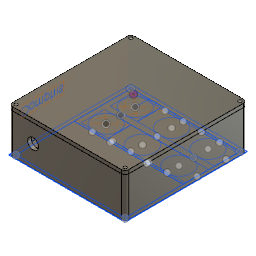
Multiple Contacts (Autodesk Fusion 360 design; units mm, degrees)
Autodesk Fusion 360 part; units mm, degrees
note: some values were not read from the file. Chosen so that the rebuilt part matches the saved one: which face or edge a step refers to; how an offset face is resized. Set by a fixed rule: which sketch regions a step uses.
sketch "Sketch1" plane through (0, 0, 0) normal (0, 1, 0) x (1, 0, 0)
  circle A0 centre (16.5, -34) radius 2.5
  line L0 (41.5, 5) -> (-8.5, 5)
  line L1 (-8.5, 5) -> (-8.5, -73)
  line L2 (-8.5, -73) -> (41.5, -73)
  line L3 (41.5, 5) -> (-8.5, -73) construction
  line L4 (-8.5, 5) -> (41.5, -73) construction
  circle A1 centre (16.5, -14) radius 17.6966
  circle A2 centre (16.5, -54.0395) radius 17.7007
  line L5 (35, 2) -> (-2, 2)
  line L6 (-2, 2) -> (-2, -30)
  line L7 (-2, -30) -> (35, -30)
  line L8 (35, -30) -> (35, 2)
  line L9 (35, 2) -> (-2, -30) construction
  line L10 (-2, 2) -> (35, -30) construction
  line L11 (35, -38.0395) -> (-2, -38.0395)
  line L12 (-2, -38.0395) -> (-2, -70.0395)
  line L13 (-2, -70.0395) -> (35, -70.0395)
  line L14 (35, -70.0395) -> (35, -38.0395)
  line L15 (35, -38.0395) -> (-2, -70.0395) construction
  line L16 (-2, -38.0395) -> (35, -70.0395) construction
  line L17 (41.5, 5) -> (91.5, 5)
  line L18 (91.5, -73) -> (41.5, -73)
  line L19 (91.5, 5) -> (141.5, 5)
  line L20 (141.5, 5) -> (141.5, -73)
  line L21 (141.5, -73) -> (91.5, -73)
  line L22 (35, 2) -> (141.5, 2)
  line L23 (141.5, 2) -> (141.5, -30)
  line L24 (141.5, -30) -> (35, -30)
  line L25 (35, -30) -> (35, 2)
  line L26 (141.5, -70.0395) -> (35, -70.0395)
  line L27 (35, -70.0395) -> (35, -38.0395)
  line L28 (35, -38.0395) -> (141.5, -38.0395)
  line L29 (141.5, -38.0395) -> (141.5, -70.0395)
  line L30 (141.5, -54.0395) -> (141.5, -73)
  line L31 (141.5, -73) -> (16.5, -73)
  line L32 (141.5, -14) -> (141.5, 5)
  line L33 (141.5, 5) -> (16.5, 5)
  line L34 (16.5, 5) -> (16.5, -14)
  line L35 (41.5, 2) -> (66.5, 2)
  line L36 (91.5, 2) -> (116.5, 2)
  line L37 (41.5, -70.0395) -> (66.5, -70.0395)
  line L38 (91.5, -70.0395) -> (116.5, -70.0395)
  line L39 (116.5, -34) -> (116.5, -38.0395)
  line L40 (116.5, -38.0395) -> (16.5, -38.0395)
  line L41 (16.5, -38.0395) -> (16.5, -34)
  circle A3 centre (66.5, -14) radius 17.697
  circle A4 centre (116.5, -14) radius 17.697
  circle A5 centre (66.5, -54.0395) radius 17.697
  circle A6 centre (116.5, -54.0395) radius 17.697
  circle A7 centre (66.5, -34) radius 2.5
  circle A8 centre (116.5, -34) radius 2.5
  line L42 (-8.5, -73) -> (141.5, -73)
  line L43 (141.5, -73) -> (141.5, -153)
  line L44 (141.5, -153) -> (-8.5, -153)
  line L45 (-8.5, -153) -> (-8.5, -73)
  line L46 (141.5, 5) -> (146.5, 5)
  line L47 (146.5, 5) -> (146.5, -153)
  line L48 (146.5, -153) -> (141.5, -153)
  line L49 (141.5, -153) -> (141.5, 5)
  line L50 (-8.5, 5) -> (-13.5, 5)
  line L51 (-13.5, 5) -> (-13.5, -153)
  line L52 (-13.5, -153) -> (-8.5, -153)
  line L53 (-8.5, -153) -> (-8.5, 5)
  line L54 (-13.5, -153) -> (146.5, -153)
  line L55 (146.5, -153) -> (146.5, -158)
  line L56 (146.5, -158) -> (-13.5, -158)
  line L57 (-13.5, -158) -> (-13.5, -153)
  line L58 (146.5, 5) -> (-13.5, 5)
  line L59 (-13.5, 5) -> (-13.5, 10)
  line L60 (-13.5, 10) -> (146.5, 10)
  line L61 (146.5, 10) -> (146.5, 5)
  circle A9 centre (-8.5, -153) radius 2.5
  circle A10 centre (-8.5, -153) radius 5
  circle A11 centre (141.5, -153) radius 2.5
  circle A12 centre (141.5, -153) radius 5
  circle A13 centre (141.5, 5) radius 2.5
  circle A14 centre (141.5, 5) radius 5
  circle A15 centre (-8.5, 5) radius 2.5
  circle A16 centre (-8.5, 5) radius 5
  point P0 (16.5, -34)
  point P1 (16.5, -14)
  point P2 (16.5, -54.0395)
  dimension "d3" = 5
  dimension "d7" = 50
  dimension "d8" = 78
  dimension "d9" = 37
  dimension "d10" = 32
  dimension "d11" = 37
  dimension "d12" = 32
  dimension "d15" = 50
  dimension "d16" = 50
  dimension "d17" = 25
  dimension "d18" = 25
  dimension "d19" = 35.394
  dimension "d20" = 35.394
  dimension "d21" = 35.394
  dimension "d22" = 35.394
  dimension "d23" = 5
  dimension "d24" = 5
  dimension "d25" = 80
  dimension "d26" = 5
  dimension "d27" = 5
  dimension "d28" = 5
  dimension "d29" = 5
  dimension "d30" = 5
  dimension "d31" = 10
  dimension "d32" = 5
  dimension "d33" = 10
  dimension "d34" = 5
  dimension "d35" = 10
  dimension "d36" = 5
  dimension "d37" = 10
  measures "d3" diameter of A0
  measures "d7" distance of L1.end L2.end
  measures "d8" distance of L0.end L1.end
  measures "d9" distance of L6.end L7.end
  measures "d10" distance of L5.end L6.end
  measures "d11" distance of L12.end L13.end
  measures "d12" distance of L11.end L12.end
  measures "d15" distance of L0.start L17.end
  measures "d16" distance of L17.end L19.end
  measures "d17" distance of L35.start L35.end
  measures "d18" distance of L36.start L36.end
  measures "d19" diameter of A3
  measures "d20" diameter of A4
  measures "d21" diameter of A5
  measures "d22" diameter of A6
  measures "d23" diameter of A7
  measures "d24" diameter of A8
  measures "d25" distance of L1.end L44.end
  measures "d26" distance of L19.end L46.end
  measures "d27" distance of L0.end L50.end
  measures "d28" distance of L51.end L56.end
  measures "d29" distance of L46.end L60.end
  measures "d30" diameter of A9
  measures "d31" diameter of A10
  measures "d32" diameter of A11
  measures "d33" diameter of A12
  measures "d34" diameter of A13
  measures "d35" diameter of A14
  measures "d36" diameter of A15
  measures "d37" diameter of A16
extrude "Extrude3" add sketch "Sketch1" along normal blind 55 contours L0 L17 L19 L33 L58 L60 A14 A16 | L0 L1 L53 L58 A15 A16 | L0 L50 L58 A15 A16 | L1 L50 L53 L58 A15 A16 | L1 L45 L51 L53 A10 A16 | L20 L23 L29 L30 L32 L43 L47 L49 A12 A14 | L19 L33 L46 L58 A13 A14 | L19 L20 L22 L32 L33 L49 L58 A13 A14 | L20 L22 L23 L32 L49 A14 | L20 L23 L32 L46 L49 L58 A13 A14 | L45 L52 L53 L54 A9 A10 | L44 L52 L54 A9 A10 | L44 L45 L53 L54 A9 A10 | L44 L48 L54 A11 A12 | L43 L48 L49 L54 A11 A12 | L44 L54 L56 A10 A12 | L43 L44 L49 L54 A11 A12 makes body 1
extrude "Extrude2" add sketch "Sketch1" along normal blind 5 separate body contours A0 A1 A2 L7 L11 L24 L28 L40 A3 A5 A7 | A0 A1 L7 | A0 A2 L11 L40 L41 | A0 L0 L1 L2 A1 A2 L5 L6 L7 L11 L12 L13 L18 L20 L21 L26 L30 L31 L34 L37 L38 A5 A6 L42 L49 L53 L58 A16 | A1 L5 L7 L8 L25 | A0 A2 L11 L41 | A2 L11 L13 L14 L27 L40 | A1 L5 L6 L7 | L8 L22 L24 L25 L35 A3 | L14 L26 L27 L28 L37 L40 A5 | A2 L11 L12 L13 | A1 L5 L34 | A1 L5 L34 | L0 A1 L5 L17 L19 L22 L33 L34 L35 L36 A3 A4 L58 A14 | L24 A3 A7 | A2 L13 | L28 L40 A5 A7 | L22 L24 L36 A3 A4 | L24 L28 L40 A3 A4 A5 A6 A7 A8 | L22 L35 A3 | L26 L28 L38 L40 A5 A6 | L26 L37 A5 | L0 L17 L19 L33 L58 L60 A14 A16 | L24 A4 A8 | L28 L39 L40 A6 A8 | L0 L1 L53 L58 A15 A16 | L0 L50 L58 A15 A16 | L20 L22 L23 L24 L32 A4 L49 A14 | L20 L24 L28 A4 A6 A8 L49 | L22 L36 A4 | L28 L39 A6 A8 | L26 L38 A6 | L0 L1 L53 L58 A15 | L0 L50 L58 A15 | L1 L50 L53 L58 A15 A16 | L1 L45 L51 L53 A10 A16 | L20 L23 L29 L30 L32 L43 L47 L49 A12 A14 | L20 L26 L28 L29 L30 A6 L49 | L19 L33 L46 L58 A13 A14 | L19 L20 L22 L32 L33 L49 L58 A13 A14 | L1 L50 L53 L58 A15 | L2 L18 L21 L31 L42 L43 L44 L45 L49 L53 L54 A10 A12 | L20 L22 L23 L32 L49 A14 | L19 L33 L46 L58 A13 | L19 L20 L32 L33 L49 L58 A13 | L20 L23 L32 L46 L49 L58 A13 A14 | L45 L52 L53 L54 A9 A10 | L44 L52 L54 A9 A10 | L44 L45 L53 L54 A9 A10 | L20 L32 L46 L49 L58 A13 | L44 L48 L54 A11 A12 | L43 L48 L49 L54 A11 A12 | L45 L52 L53 L54 A9 | L44 L52 L54 A9 | L44 L54 L56 A10 A12 | L44 L45 L53 L54 A9 | L43 L44 L49 L54 A11 A12 | L44 L48 L54 A11 | L43 L48 L49 L54 A11 | L43 L44 L49 L54 A11 makes body 2
extrude "Extrude1" add sketch "Sketch1" along normal blind 5 separate body contours A0 A1 A2 | A0 A1 A2 L7 L11 L24 L28 L40 A3 A5 A7 | A0 A1 L7 | A0 A2 L11 L40 L41 | A0 L0 L1 L2 A1 A2 L5 L6 L7 L11 L12 L13 L18 L20 L21 L26 L30 L31 L34 L37 L38 A5 A6 L42 L49 L53 L58 A16 | A1 L5 L7 | A1 L5 L7 L8 L25 | A0 A2 L11 L41 | A2 L11 L13 L14 L27 L40 | A2 L11 L13 L40 | A1 L5 L6 L7 | A2 L11 L12 L13 | A1 L5 L34 | A1 L5 L34 | L0 A1 L5 L17 L19 L22 L33 L34 L35 L36 A3 A4 L58 A14 | A2 L13 makes body 3
sketch "Sketch2" plane through (0, 0, 158) normal (0, 0, 1) x (1, 0, 0)
  line L0 (-8.5, 0) -> (141.5, 0)
  line L1 (141.5, 0) -> (141.5, 55)
  line L2 (141.5, 55) -> (-8.5, 55)
  line L3 (-8.5, 55) -> (-8.5, 0)
  circle A0 centre (20, 30) radius 7.4912
extrude "Extrude4" cut sketch "Sketch2" against normal blind 20 contours A0 bodies 1
combine "Combine1" operation add target body 1 tool bodies 2
extrude "Extrude5" add sketch "Sketch1" along normal blind 5 separate body contours A0 A1 A2 | A0 A1 A2 L7 L11 L24 L28 L40 A3 A5 A7 | A0 A1 | A0 A1 L7 | A0 A2 L11 L40 L41 | A0 A2 L41 | A0 L0 L1 L2 A1 A2 L5 L6 L7 L11 L12 L13 L18 L20 L21 L26 L30 L31 L34 L37 L38 A5 A6 L42 L49 L53 L58 A16 | A1 L5 L7 | A1 L5 L7 L8 L25 | A0 A2 L11 L41 | A0 A2 L41 | A2 L11 L13 L14 L27 L40 | A2 L11 L13 L40 | A1 L5 L6 L7 | L8 L22 L24 L25 L35 A3 | L14 L26 L27 L28 L37 L40 A5 | A2 L11 L12 L13 | A1 L5 L34 | A1 L5 L34 | L0 A1 L5 L17 L19 L22 L33 L34 L35 L36 A3 A4 L58 A14 | L22 L24 L35 A3 | L24 A3 A7 | A2 L13 | L28 L40 A5 A7 | L26 L28 L37 L40 A5 | L22 L24 L36 A3 A4 | L24 L28 L40 A3 A4 A5 A6 A7 A8 | L22 L35 A3 | A3 A7 | A3 A5 A7 | L26 L28 L38 L40 A5 A6 | A5 A7 | L26 L37 A5 | L0 L17 L19 L33 L58 L60 A14 A16 | L22 L24 L36 A4 | L24 A4 A8 | L28 L39 L40 A6 A8 | L26 L28 L38 L40 A6 | L0 L1 L53 L58 A15 A16 | L0 L50 L58 A15 A16 | L20 L22 L23 L24 L32 A4 L49 A14 | L20 L24 L28 A4 A6 A8 L49 | L22 L36 A4 | A4 A8 | A4 A6 A8 | L28 L39 A6 A8 | L39 A6 A8 | L26 L38 A6 | L1 L50 L53 L58 A15 A16 | L1 L45 L51 L53 A10 A16 | L20 L23 L29 L30 L32 L43 L47 L49 A12 A14 | L20 L26 L28 L29 L30 A6 L49 | L39 A6 A8 | L19 L33 L46 L58 A13 A14 | L19 L20 L22 L32 L33 L49 L58 A13 A14 | L2 L18 L21 L31 L42 L43 L44 L45 L49 L53 L54 A10 A12 | L20 L22 L23 L32 L49 A14 | L20 L23 L32 L46 L49 L58 A13 A14 | L45 L52 L53 L54 A9 A10 | L44 L52 L54 A9 A10 | L44 L45 L53 L54 A9 A10 | L44 L48 L54 A11 A12 | L43 L48 L49 L54 A11 A12 | L44 L54 L56 A10 A12 | L43 L44 L49 L54 A11 A12 makes body 4
move_body "Move1" bodies 4 to x (1, 0, 0) y (0, 1, 0) z (0, 0, 1) at (0, 55, 0)
thread "Thread1" "ISO Metric profile 5.0 M5x0.8 6H" major diameter 5.12 minor diameter 4.234 pitch 0.8 angle 60 resizes the face on face at (142.2962, 21.6667, 150.6302) on bodies 1
thread "Thread2" "ISO Metric profile 5.0 M5x0.8 6H" major diameter 5.12 minor diameter 4.234 pitch 0.8 angle 60 resizes the face on face at (142.0894, 58.3333, 150.5705) on bodies 4
thread "Thread3" "ISO Metric profile 5.0 M5x0.8 6H" major diameter 5.12 minor diameter 4.234 pitch 0.8 angle 60 resizes the face on face at (142.2962, 56.6667, -7.3698) on bodies 4
thread "Thread4" "ISO Metric profile 5.0 M5x0.8 6H" major diameter 5.12 minor diameter 4.234 pitch 0.8 angle 60 resizes the face on face at (142.1771, 21.6667, -2.5934) on bodies 1
thread "Thread5" "ISO Metric profile 5.0 M5x0.8 6H" major diameter 5.12 minor diameter 4.234 pitch 0.8 angle 60 resizes the face on face at (-6.0031, 21.6667, -5.1246) on bodies 1
thread "Thread6" "ISO Metric profile 5.0 M5x0.8 6H" major diameter 5.12 minor diameter 4.234 pitch 0.8 angle 60 resizes the face on face at (-6.0124, 58.3333, -5.2489) on bodies 4
thread "Thread7" "ISO Metric profile 5.0 M5x0.8 6H" major diameter 5.12 minor diameter 4.234 pitch 0.8 angle 60 resizes the face on face at (-6.0496, 21.6667, 152.5046) on bodies 1
thread "Thread8" "ISO Metric profile 5.0 M5x0.8 6H" major diameter 5.12 minor diameter 4.234 pitch 0.8 angle 60 resizes the face on face at (-6.0773, 58.3333, 152.3831) on bodies 4
sketch "Sketch4" plane through (-13.5, 0, 0) normal (-1, 0, 0) x (0, 0, 1)
  line L0 (153, 0) -> (153, 55)
  line L1 (153, 55) -> (-5, 55)
  line L2 (-5, 55) -> (-5, 0)
  line L3 (-5, 0) -> (153, 0)
  line L4 (140, 50) -> (82.5488, 50) construction
  line L5 (82.5488, 50) -> (82.5488, 35) construction
  line L6 (82.5488, 35) -> (140, 35) construction
  line L7 (140, 35) -> (140, 50) construction
hidden bodies 3
equation "d19 = ( 17.697 * 2 ) * 1 mm"
named bodies: "Test", "Top", "Bottom"
